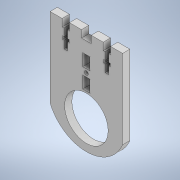
# Autodesk Inventor part: Крепление_мотора2_платформа
Saved by Autodesk Inventor 2020 (Build 240168000, 168)
## iProperties
Created: 2022-02-01
Part Number: Крепление_мотора2_платформа
Material: Типовые
Document SubType Name: Modeling
Designer: Администратор
Density: 1 g/cm^3
Appearance: По умолчанию
Autodesk Inventor part; units mm, degrees
ref_plane "YZ Plane" through (0, 0, 0) normal (1, 0, 0) x (0, 1, 0)
ref_plane "XZ Plane" through (0, 0, 0) normal (0, 1, 0) x (-1, 0, 0)
ref_plane "XY Plane" through (0, 0, 0) normal (0, 0, 1) x (1, 0, 0)
sketch "0" plane through (0, 0, 0) normal (0, 0, 1) x (1, 0, 0)
  line L0 (4, 47) -> (4, 53)
  line L1 (4, 53) -> (14, 53)
  line L2 (14, 53) -> (14, 47)
  line L3 (20, 47) -> (18.5, 47)
  line L4 (18.5, 47) -> (18.5, 40.75)
  line L5 (18.5, 32) -> (15.5, 32)
  line L6 (15.5, 32) -> (15.5, 38.25)
  line L7 (14.25, 40.75) -> (15.5, 40.75)
  line L8 (19.75, 40.75) -> (19.75, 38.25)
  line L9 (19.75, 38.25) -> (18.5, 38.25)
  line L10 (14.25, 38.25) -> (14.25, 40.75)
  line L11 (15.5, 40.75) -> (15.5, 47)
  line L12 (15.5, 38.25) -> (14.25, 38.25)
  line L13 (18.5, 40.75) -> (19.75, 40.75)
  line L14 (15.5, 47) -> (14, 47)
  line L15 (20, 53) -> (30, 53)
  line L16 (20, 47) -> (20, 53)
  line L17 (18.5, 38.25) -> (18.5, 32)
  line L18 (-30, 53) -> (-20, 53)
  line L19 (-20, 53) -> (-20, 47)
  line L20 (-14, 47) -> (-15.5, 47)
  line L21 (-15.5, 47) -> (-15.5, 40.75)
  line L22 (-15.5, 32) -> (-18.5, 32)
  line L23 (-18.5, 32) -> (-18.5, 38.25)
  line L24 (-19.75, 40.75) -> (-18.5, 40.75)
  line L25 (-14.25, 40.75) -> (-14.25, 38.25)
  line L26 (-14.25, 38.25) -> (-15.5, 38.25)
  line L27 (-19.75, 38.25) -> (-19.75, 40.75)
  line L28 (-18.5, 40.75) -> (-18.5, 47)
  line L29 (-18.5, 38.25) -> (-19.75, 38.25)
  line L30 (-15.5, 40.75) -> (-14.25, 40.75)
  line L31 (-18.5, 47) -> (-20, 47)
  line L32 (-14, 53) -> (-4, 53)
  line L33 (-14, 47) -> (-14, 53)
  line L34 (-4, 53) -> (-4, 47)
  line L35 (-15.5, 38.25) -> (-15.5, 32)
  line L36 (-3, 47) -> (-4, 47)
  line L37 (3, 47) -> (4, 47)
  line L38 (30, 53) -> (30, 47)
  circle A0 centre (0, -8.5) radius 18
  line L39 (30, 47) -> (30, -12.5)
  line L40 (-30, -12.5) -> (-30, 53)
  arc A1 (-30, -12.5) -> (30, -12.5) centre (0, 0) ccw
  line L41 (-3, 11) -> (-3, 21)
  line L42 (-3, 21) -> (3, 21)
  line L43 (3, 21) -> (3, 11)
  line L44 (3, 11) -> (-3, 11)
  line L45 (-3, 27) -> (-3, 37)
  line L46 (3, 37) -> (3, 27)
  line L47 (3, 27) -> (-3, 27)
  circle A2 centre (0, 24) radius 1.6
  line L48 (-3, 37) -> (3, 37)
  line L49 (-3, 47) -> (3, 47)
  point P0 (30, -12.5)
  constraints: 100 end point, 3 centre point, 2 point on circle
extrude "Выдавливание1" add sketch "0" along normal blind 6
